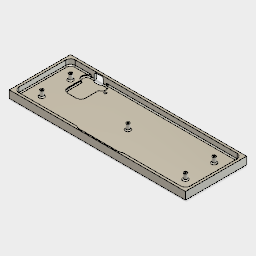
bottom (Autodesk Fusion 360 design; units mm, degrees)
Autodesk Fusion 360 part; units mm, degrees
sketch "Sketch1" plane through (0, 0, 0) normal (0, 1, 0) x (1, 0, 0)
  line L0 (0, 0) -> (233, 0)
  line L1 (233, 0) -> (233, -81)
  line L2 (233, -81) -> (0, -81)
  line L3 (0, -81) -> (0, 0)
  circle A0 centre (59.5, -13.5) radius 2.75
  point P0 (59.5, -13.5)
  dimension "d1" = 233
  dimension "d2" = 81
  dimension "d59" = 5.5
  measures "d1" distance of L0.start L0.end
  measures "d2" distance of L0.start L2.end
  measures "d59" diameter of A0
extrude "Extrude1" add sketch "Sketch1" along normal blind 11.5 contours L0 L1 L2 L3 | A0
sketch "Sketch2" plane through (0, 11.5, 0) normal (0, 1, 0) x (-1, 0, 0)
  line L0 (0, 81) -> (-233, 81)
  line L1 (-233, 81) -> (-233, 0)
  line L2 (-233, 0) -> (0, 0)
  line L3 (0, 0) -> (0, 81)
  line L4 (-3.1, 71.55) -> (-3.1, 9.45)
  line L5 (-9.45, 3.1) -> (-223.55, 3.1)
  line L6 (-229.9, 9.45) -> (-229.9, 71.55)
  line L7 (-223.55, 77.9) -> (-9.45, 77.9)
  arc A0 (-9.45, 3.1) -> (-3.1, 9.45) centre (-9.45, 9.45) ccw
  arc A1 (-229.9, 9.45) -> (-223.55, 3.1) centre (-223.55, 9.45) ccw
  arc A2 (-223.55, 77.9) -> (-229.9, 71.55) centre (-223.55, 71.55) ccw
  arc A3 (-3.1, 71.55) -> (-9.45, 77.9) centre (-9.45, 71.55) ccw
  line L8 (-86.25, 79.55) -> (-146.75, 79.55)
  line L9 (-146.75, 79.55) -> (-146.75, 77.9)
  line L10 (-146.75, 77.9) -> (-86.25, 77.9)
  line L11 (-86.25, 77.9) -> (-86.25, 79.55)
  dimension "d8" = 6.35
  dimension "d9" = 6.35
  dimension "d10" = 6.35
  dimension "d11" = 6.35
  dimension "d86" = 60.5
  measures "d8" radius of A0
  measures "d9" radius of A1
  measures "d10" radius of A2
  measures "d11" radius of A3
  measures "d86" distance of L8.start L8.end
extrude "Extrude12" cut sketch "Sketch2" against normal blind 4.35 contours L7 L8 L9 L10 L11
extrude "Extrude2" cut sketch "Sketch2" against normal blind 7.5 contours L4 L5 L6 L7 A0 A1 A2 A3 L10
sketch "Sketch3" plane through (0, 0, 0) normal (0, 0, 1) x (1, 0, 0)
  line L0 (44.4, 10) -> (36.6, 10)
  arc A0 (46.4, 8) -> (44.4, 10) centre (44.4, 8) ccw
  arc A1 (36.6, 10) -> (34.6, 8) centre (36.6, 8) ccw
  line L1 (46.4, -0.05) -> (46.4, 8)
  line L2 (34.6, -0.05) -> (34.6, 8)
  line L3 (46.4, -0.05) -> (34.6, -0.05)
  point P0 (34.6, 10)
  dimension "d17" = 2
  dimension "d18" = 2
  measures "d17" radius of A0
  measures "d18" radius of A1
extrude "Extrude3" cut sketch "Sketch3" along normal blind 3.1
sketch "Sketch4" plane through (0, 4, 0) normal (0, 1, 0) x (-1, 0, 0)
  arc A0 (-9.45, 3.1) -> (-3.1, 9.45) centre (-9.45, 9.45) ccw
  line L0 (-3.1, 9.45) -> (-3.1, 71.55)
  arc A1 (-3.1, 71.55) -> (-9.45, 77.9) centre (-9.45, 71.55) ccw
  line L1 (-9.45, 77.9) -> (-223.55, 77.9)
  arc A2 (-223.55, 77.9) -> (-229.9, 71.55) centre (-223.55, 71.55) ccw
  line L2 (-229.9, 71.55) -> (-229.9, 9.45)
  arc A3 (-229.9, 9.45) -> (-223.55, 3.1) centre (-223.55, 9.45) ccw
  line L3 (-223.55, 3.1) -> (-46.4, 3.1)
  line L4 (-46.4, 3.1) -> (-34.6, 3.1)
  line L5 (-34.6, 3.1) -> (-9.45, 3.1)
  circle A4 centre (-59.5, 13.5) radius 1.5
  line L6 (-34.95, 38.8) -> (-46.05, 38.8)
  arc A5 (-28.6, 32.45) -> (-34.95, 38.8) centre (-34.95, 32.45) ccw
  arc A6 (-46.05, 38.8) -> (-52.4, 32.45) centre (-46.05, 32.45) ccw
  arc A7 (-52.4, 15.4768) -> (-50.4, 3.1) centre (-50.4, 9.45) ccw
  arc A8 (-30.6, 3.1) -> (-28.6, 15.4768) centre (-30.6, 9.45) ccw
  line L7 (-28.6, 15.4768) -> (-28.6, 32.45)
  line L8 (-52.4, 15.4768) -> (-52.4, 32.45)
  line L9 (-34.6, 3.1) -> (-46.4, 3.1)
  line L10 (-46.4, 3.1) -> (-46.4, 2.825)
  line L11 (-43.225, 6) -> (-37.775, 6)
  line L12 (-34.6, 2.825) -> (-34.6, 3.1)
  line L13 (-30.6, 3.1) -> (-34.6, 3.1)
  line L14 (-46.4, 3.1) -> (-50.4, 3.1)
  arc A9 (-34.6, 2.825) -> (-37.775, 6) centre (-37.775, 2.825) ccw
  arc A10 (-43.225, 6) -> (-46.4, 2.825) centre (-43.225, 2.825) ccw
  circle A11 centre (-116.5, 40.5) radius 2.225
  circle A12 centre (-211.5, 21.5) radius 2.225
  circle A13 centre (-211.5, 59.5) radius 2.225
  circle A14 centre (-21.5, 59.5) radius 2.225
  circle A15 centre (-21.5, 21.5) radius 2.225
  point P0 (-59.5, 13.5)
  point P1 (-28.6, 38.8)
  point P2 (-52.4, 38.8)
  point P3 (-21.5, 59.5)
  point P4 (-211.5, 59.5)
  point P5 (-211.5, 21.5)
  point P6 (-116.5, 40.5)
  dimension "d22" = 3
  dimension "d28" = 23.8
  dimension "d30" = 6.35
  dimension "d31" = 6.35
  dimension "d33" = 4
  dimension "d37" = 3.175
  dimension "d38" = 3.175
  dimension "d43" = 4.45
  dimension "d44" = 4.45
  dimension "d45" = 4.45
  dimension "d46" = 4.45
  dimension "d47" = 4.45
  measures "d22" diameter of A4
  measures "d28" distance of P1 P2
  measures "d30" radius of A5
  measures "d31" radius of A6
  measures "d33" distance of L3.end A7.end
  measures "d37" radius of A9
  measures "d38" radius of A10
  measures "d43" diameter of A11
  measures "d44" diameter of A12
  measures "d45" diameter of A13
  measures "d46" diameter of A14
  measures "d47" diameter of A15
extrude "Extrude5" cut sketch "Sketch4" against normal blind 2.5 contours L3 L4 L5 L6 A5 A6 A7 A8 L7 L8 L9 L11 L13 L14 A9 A10
extrude "Extrude4" cut sketch "Sketch4" against normal blind 4 contours A4
extrude "Extrude6" cut sketch "Sketch4" against normal blind 4 contours L4 L9 L11 A9 A10
extrude "Extrude7" add sketch "Sketch4" along normal up to surface (7.5 mm away) contours A12
extrude "Extrude8" add sketch "Sketch4" along normal up to surface (7.5 mm away) contours A13
extrude "Extrude9" add sketch "Sketch4" along normal up to surface (7.5 mm away) contours A11
extrude "Extrude10" add sketch "Sketch4" along normal up to surface (7.5 mm away) contours A15
extrude "Extrude11" add sketch "Sketch4" along normal up to surface (7.5 mm away) contours A14
chamfer "Chamfer1" distance 1.5 angle 45 5 edges at (139.7, 0, 0) (17.3, 0, 0) (0, 0, 40.5) (116.5, 0, 81) (233, 0, 40.5)
chamfer "Chamfer2" distance 1.25 angle 49 1 edges at (60.8985, 0, 12.9576) measured on face at (174.6422, 0, 31.6545)
fillet "Fillet1" radius 1.27 9 edges at (136.975, 4, 3.1) (228.0401, 4, 4.9599) (229.9, 4, 40.5) (228.0401, 4, 76.0401) (116.5, 4, 77.9) (4.9599, 4, 76.0401) (3.1, 4, 40.5) (4.9599, 4, 4.9599) (20.025, 4, 3.1)
fillet "Fillet2" radius 1.27 1 edges at (118.5744, 4, 41.3046)
fillet "Fillet3" radius 1.27 1 edges at (213.5744, 4, 22.3046)
fillet "Fillet4" radius 1.27 1 edges at (213.5744, 4, 60.3046)
fillet "Fillet5" radius 1.27 1 edges at (23.5744, 4, 22.3046)
fillet "Fillet6" radius 1.27 1 edges at (23.5744, 4, 60.3046)
fillet "Fillet7" radius 1.27 9 edges at (24.3313, 1.5, 8.437) (32.6, 1.5, 3.1) (52.4, 1.5, 23.9634) (50.5401, 1.5, 36.9401) (40.5, 1.5, 38.8) (30.4599, 1.5, 36.9401) (28.6, 1.5, 23.9634) (48.4, 1.5, 3.1) (56.6687, 1.5, 8.437)
hole "Hole1" at (21.5, 11.5, 59.5) direction (0, -1, 0) diameter 2 depth 6 tip angle 118
hole "Hole2" at (21.5, 11.5, 21.5) direction (0, -1, 0) diameter 2 depth 6 tip angle 118
hole "Hole3" at (116.5, 11.5, 40.5) direction (0, -1, 0) diameter 2 depth 6 tip angle 118
hole "Hole4" at (211.5, 11.5, 59.5) direction (0, -1, 0) diameter 2 depth 6 tip angle 118
hole "Hole5" at (211.5142, 11.5, 21.4921) direction (0, -1, 0) diameter 2 depth 6 tip angle 118
fillet "Fillet8" radius 6.35 1 edges at (146.75, 9.325, 79.55)
fillet "Fillet9" radius 6.35 1 edges at (86.25, 9.325, 79.55)
fillet "Fillet10" radius 1.27 3 edges at (88.2311, 7.15, 79.1232) (116.5, 7.15, 79.55) (144.7689, 7.15, 79.1232)
